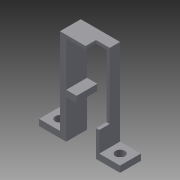
# Autodesk Inventor part: MotorMount
Saved by Autodesk Inventor 2014 SP1 (Build 180222100, 222)
## iProperties
Created: 2014-06-07
Part Number: MotorMount
Material: Generic
Document SubType Name: Modeling
Designer: Erin
Density: 1 g/cm^3
Appearance: Default
Author: Erin
Autodesk Inventor part; units mm, degrees
ref_plane "YZ Plane" through (0, 0, 0) normal (1, 0, 0) x (0, 1, 0)
ref_plane "XZ Plane" through (0, 0, 0) normal (0, 1, 0) x (-1, 0, 0)
ref_plane "XY Plane" through (0, 0, 0) normal (0, 0, 1) x (1, 0, 0)
sketch "Sketch1" plane through (0, 0, 0) normal (0, 1, 0) x (-1, 0, 0)
  line L0 (-9.45, 13.9) -> (9.45, 13.9)
  line L1 (9.45, 13.9) -> (9.45, 12.4)
  line L2 (9.45, 12.4) -> (-9.45, 12.4)
  line L3 (-9.45, 12.4) -> (-9.45, 13.9)
  line L4 (9.45, 12.4) -> (6.45, 12.4)
  line L5 (6.45, 12.4) -> (6.45, -9)
  line L6 (6.45, -9) -> (9.45, -9)
  line L7 (9.45, -9) -> (9.45, 12.4)
  line L8 (-9.45, 12.4) -> (-7.95, 12.4)
  line L9 (-7.95, 12.4) -> (-7.95, -9)
  line L10 (-7.95, -9) -> (-9.45, -9)
  line L11 (-9.45, -9) -> (-9.45, 12.4)
  line L12 (-7.95, -7.6) -> (-9.45, -7.6)
  line L13 (-9.45, -7.6) -> (-9.45, -10.6)
  line L14 (-9.45, -10.6) -> (-7.95, -10.6)
  line L15 (-7.95, -10.6) -> (-7.95, -7.6)
  line L16 (1.45, -9) -> (9.45, -9)
  line L17 (9.45, -9) -> (9.45, -12)
  line L18 (9.45, -12) -> (1.45, -12)
  line L19 (1.45, -12) -> (1.45, -9)
  line L20 (-9.45, -10.6) -> (-7.95, -10.6)
  line L21 (-7.95, -10.6) -> (-7.95, -27.6)
  line L22 (-7.95, -27.6) -> (-9.45, -27.6)
  line L23 (-9.45, -27.6) -> (-9.45, -10.6)
  line L24 (9.45, -12) -> (6.45, -12)
  line L25 (6.45, -12) -> (6.45, -27.6)
  line L26 (6.45, -27.6) -> (9.45, -27.6)
  line L27 (9.45, -27.6) -> (9.45, -12)
  line L28 (-7.95, -27.6) -> (-19.45, -27.6)
  line L29 (-19.45, -27.6) -> (-19.45, -30.6)
  line L30 (-19.45, -30.6) -> (-7.95, -30.6)
  line L31 (-7.95, -30.6) -> (-7.95, -27.6)
  line L32 (6.45, -27.6) -> (19.45, -27.6)
  line L33 (19.45, -27.6) -> (19.45, -30.6)
  line L34 (19.45, -30.6) -> (6.45, -30.6)
  line L35 (6.45, -30.6) -> (6.45, -27.6)
  line L36 (-14.45, -26) -> (-14.45, -42) construction
  line L37 (14.45, -27) -> (14.45, -42) construction
  point P0 (0, 0)
  point P1 (0, 12.4)
  dimension "d0" = 1.5
  dimension "d1" = 3
  dimension "d2" = 1.5
  dimension "d3" = 3
  dimension "d4" = 3
  dimension "d5" = 0
  dimension "d6" = 5
  dimension "d7" = 14.4
  dimension "d8" = 21.4
  dimension "d9" = 20
  dimension "d12" = 0
  dimension "d13" = 0
  dimension "d20" = 17
  dimension "d21" = 10
  dimension "d22" = 1.5
  dimension "d23" = 3
  dimension "d24" = 10
  dimension "d25" = 3
  dimension "d26" = 3
  dimension "d33" = 5
  dimension "d34" = 5
  dimension "d35" = 28.9
  constraints: 76 end point, 20 parallel, 9 horizontal, 9 perpendicular, 2 collinear, 1 midpoint, 1 vertical alignment
  measures "d0" distance of L0.end L1.end
  measures "d1" distance of L5.end L6.end
  measures "d2" distance of L9.end L10.end
  measures "d3" distance of L14.end L12.start
  measures "d4" distance of L18.end L16.start
  measures "d5" distance between parallel lines of L15 L9
  measures "d6" distance between parallel lines of L5 L19
  measures "d7" distance between parallel lines of L5 L9
  measures "d8" distance between parallel lines of L16 L2
  measures "d9" distance between parallel lines of L12 L2
  measures "d12" distance between parallel lines of L11 L13
  measures "d13" distance between parallel lines of L7 L17
  measures "d20" distance of L22.end L13.end
  measures "d21" distance between parallel lines of L23 L29
  measures "d22" distance of L21.end L22.end
  measures "d23" distance of L25.end L26.end
  measures "d24" distance between parallel lines of L27 L33
  measures "d25" distance of L28.end L29.end
  measures "d26" distance of L32.end L33.end
  measures "d33" distance between parallel lines of L23 L36
  measures "d34" distance between parallel lines of L27 L37
  measures "d35" distance between parallel lines of L37 L36
extrude "Extrusion1" add sketch "Sketch1" along normal blind 10
sketch "Sketch6" plane through (19.45, 0, -30.6) normal (0, 0, -1) x (-1, 0, 0)
  line L0 (0, 10) -> (11.5, 10) projected
  line L1 (0, 0) -> (10, 0)
  line L2 (10, 0) -> (10, 10)
  line L3 (10, 10) -> (0, 10)
  line L4 (0, 10) -> (0, 0)
  circle A0 centre (5, 5) radius 2.25
  point P0 (19.45, 0)
  dimension "d27" = 4.5
  constraints: 8 end point, 2 parallel, 1 centre point, 1 horizontal, 1 perpendicular, 1 point on line
  measures "d27" diameter of A0
sketch "Sketch7" plane through (-6.45, 0, -30.6) normal (0, 0, -1) x (-1, 0, 0)
  line L0 (0, 10) -> (13, 10) projected
  line L1 (13, 0) -> (3, 0)
  line L2 (3, 0) -> (3, 10)
  line L3 (3, 10) -> (13, 10)
  line L4 (13, 10) -> (13, 0)
  circle A0 centre (8, 5) radius 2.25
  point P0 (-6.45, 0)
  dimension "d28" = 4.5
  constraints: 8 end point, 2 parallel, 1 centre point, 1 horizontal, 1 perpendicular, 1 point on line
  measures "d28" diameter of A0
extrude "Extrusion4" cut sketch "Sketch6" against normal blind 4 contours A0
extrude "Extrusion5" cut sketch "Sketch7" against normal blind 4 contours A0
sketch "Sketch8" plane through (0, 0, 0) normal (0, -1, 0) x (1, 0, 0)
  line L0 (2.9056, 16.2719) -> (14.45, 16.2719)
  line L1 (14.45, 16.2719) -> (14.45, -17.7657)
  line L2 (14.45, -17.7657) -> (2.9056, -17.7657)
  line L3 (2.9056, -17.7657) -> (2.9056, 16.2719)
  point P0 (0, 0)
  constraints: 8 end point, 2 parallel, 1 horizontal, 1 perpendicular
extrude "Extrusion6" cut sketch "Sketch8" against normal blind 5
equation "\"sp\" = 0.4"
body "Solid1"
